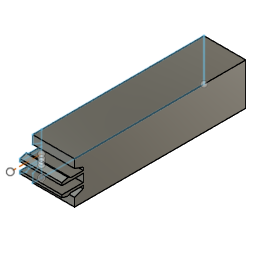
conveyor-spacer (Autodesk Fusion 360 design; units mm, degrees)
Autodesk Fusion 360 part; units mm, degrees
sketch "Sketch1" plane through (0, 0, 0) normal (1, 0, 0) x (0, 1, 0)
  line L0 (77.85, 0) -> (77.85, 20)
  line L1 (0, 10) -> (-14.9603, 10) construction
  line L2 (-4.15, 16) -> (0, 14.4895)
  line L3 (-7.2644, 13.9) -> (-10.25, 13.1)
  line L4 (0, 6.9) -> (-6, 6.9)
  line L5 (0, 20) -> (-4.15, 20)
  line L6 (0, 0) -> (77.85, 0)
  line L7 (-10.25, 6.9) -> (-10.25, 8.1)
  line L8 (-6, 6.9) -> (-7.2644, 6.1)
  line L9 (-10.25, 8.1) -> (0, 8.1)
  line L10 (-4.15, 4) -> (0, 5.5105)
  line L11 (-10.25, 13.1) -> (-10.25, 11.9)
  line L12 (-7.2644, 6.1) -> (-10.25, 6.9)
  line L13 (0, 10) -> (-14.9603, 10) construction
  line L14 (-4.15, 20) -> (-4.15, 16)
  line L15 (-4.15, 0) -> (-4.15, 4)
  line L16 (0, 20) -> (0, 0)
  line L17 (-6, 13.1) -> (-7.2644, 13.9)
  line L18 (0, 0) -> (-4.15, 0)
  line L19 (77.85, 0) -> (77.85, 20)
  line L20 (-10.25, 11.9) -> (0, 11.9)
  line L21 (0, 13.1) -> (-6, 13.1)
  line L22 (77.85, 20) -> (0, 20)
  dimension "d1" = 20
  dimension "d2" = 6
  dimension "d3" = 1.85
  dimension "d4" = 4
  dimension "d5" = 1.2
  dimension "d6" = 4.25
  dimension "d7" = 3.1
  dimension "d8" = 70
  dimension "d9" = 0.8
  dimension "d10" = 105
  dimension "d14" = 20
  dimension "d21" = 82
  constraint horizontal L6
  constraint vertical L0
  constraint horizontal L22
  constraint vertical L16
  constraint coincident L6.start L16.end
  constraint midpoint L1.start L16
  constraint perpendicular L13 L16
  constraint coincident L21.start L16
  constraint perpendicular L16 L21
  constraint perpendicular L11 L21
  constraint coincident L20.end L16
  constraint perpendicular L16 L20
  constraint perpendicular L5 L16
  constraint perpendicular L14 L22
  constraint coincident L2.end L16
  constraint coincident L3.end L21
  constraint symmetric L5.start L6.start L13
  constraint symmetric L1.start L13.start L13
  constraint symmetric L1.end L13.end L13
  constraint symmetric L4.start L21.start L13
  constraint symmetric L17.start L4.end L13
  constraint symmetric L8.end L3.start L13
  constraint symmetric L3.end L7.start L13
  constraint symmetric L11.end L7.end L13
  constraint symmetric L9.end L20.end L13
  constraint symmetric L5.end L15.start L13
  constraint symmetric L10.start L2.start L13
  constraint symmetric L10.end L2.end L13
  constraint vertical L19
  measures "d1" distance of L5.start L6.start
  measures "d2" distance of L17.start L21.start
  measures "d3" distance of L17.start L14
  measures "d4" distance of L5.end L2.start
  measures "d5" distance of L20 L21
  measures "d6" distance of L17.start L11
  measures "d7" distance of L13 L21
  measures "d8" angle of L2 L16
  measures "d9" distance of L3.start L21
  measures "d10" angle of L3 L11
  measures "d14" distance of L0.end L0.start
  measures "d21" distance of L0 L14
extrude "Extrude1" add sketch "Sketch1" along normal blind 20
